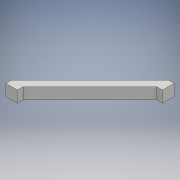
# Autodesk Inventor part: frame_rod_2
Saved by Autodesk Inventor 2017 (Build 210142000, 142)
## iProperties
Created: 2017-01-29
Part Number: frame_rod_2
Material: Generic
Document SubType Name: Modeling
Designer: Gabe Madonna
Density: 1 g/cm^3
Appearance: Default
Author: Gabe Madonna
Autodesk Inventor part; units mm, degrees
ref_plane "YZ Plane" through (0, 0, 0) normal (1, 0, 0) x (0, 1, 0)
ref_plane "XZ Plane" through (0, 0, 0) normal (0, 1, 0) x (-1, 0, 0)
ref_plane "XY Plane" through (0, 0, 0) normal (0, 0, 1) x (1, 0, 0)
sketch "Sketch1" plane through (0, 0, 0) normal (0, 0, 1) x (1, 0, 0)
  line L0 (0, 0) -> (58.0499, 58.0499)
  line L1 (0, 0) -> (82.095, 0) construction
  line L2 (58.0499, 58.0499) -> (63.0499, 58.0499)
  line L3 (63.0499, 58.0499) -> (63.0499, 68.0499)
  line L4 (63.0499, 68.0499) -> (58.0499, 68.0499)
  line L5 (0, 0) -> (0, -5)
  line L6 (0, -5) -> (-10, -5)
  line L7 (-10, -5) -> (-10, 0)
  line L8 (58.0499, 68.0499) -> (-10, 0)
  dimension "d0" = 45
  dimension "d1" = 82.095
  dimension "d2" = 5
  dimension "d3" = 10
  dimension "d4" = 5
  dimension "d5" = 5
  dimension "d6" = 10
  constraints: 18 end point, 4 perpendicular, 2 horizontal, 1 equal length, 1 parallel, 1 vertical
  measures "d0" angle of L1 L0
  measures "d1" distance of L0.start L0.end
  measures "d2" distance of L0.end L2.end
  measures "d3" distance of L2.end L3.end
  measures "d4" distance of L3.end L4.end
  measures "d5" distance of L0.start L5.end
  measures "d6" distance of L5.end L6.end
extrude "Extrusion1" add sketch "Sketch1" along normal blind 10
body "Solid1"
